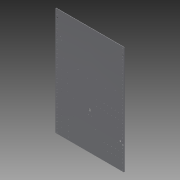
# Autodesk Inventor part: Electronics plate
Saved by Autodesk Inventor 2015 (Build 190159000, 159)
## iProperties
Created: 2015-01-17
Part Number: Electronics plate
Material: Generic
Document SubType Name: Modeling
Designer: chapale16
Density: 1 g/cm^3
Appearance: Default
Author: chapale16
Autodesk Inventor part; units mm, degrees
ref_plane "YZ Plane" through (0, 0, 0) normal (1, 0, 0) x (0, 1, 0)
ref_plane "XZ Plane" through (0, 0, 0) normal (0, 1, 0) x (-1, 0, 0)
sketch "Sketch2" plane through (0, 0, 0) normal (0, 0, 1) x (1, 0, 0)
  line L0 (0, 0) -> (566.42, 0)
  line L1 (566.42, 0) -> (566.42, -1727.2)
  line L2 (566.42, -1727.2) -> (0, -1727.2)
  line L3 (0, -1727.2) -> (0, 0)
  dimension "d0" = 566.42
  dimension "d1" = 1727.2
  constraints: 8 end point, 2 parallel, 1 horizontal, 1 perpendicular
  measures "d0" distance of L1.end L2.end
  measures "d1" distance of L0.end L1.end
extrude "Extrusion1" add sketch "Sketch2" along normal blind 3.175
sketch "Sketch4" plane through (0, 0, 3.175) normal (0, 0, 1) x (1, 0, 0)
  line L0 (566.42, 0) -> (0, 0) projected
  line L1 (0, 0) -> (0, -1727.2) projected
  line L2 (0, -1727.2) -> (566.42, -1727.2) projected
  line L3 (566.42, -1727.2) -> (566.42, 0) projected
  line L4 (0, -1727.2) -> (566.42, -1727.2) projected
  line L5 (68.58, -1727.2) -> (500.38, -1727.2)
  circle A0 centre (68.58, -1391.92) radius 12.7
  circle A1 centre (500.38, -1391.92) radius 12.7
  circle A2 centre (68.58, -1727.2) radius 12.7
  circle A3 centre (500.38, -1727.2) radius 12.7
  dimension "d6" = 25.4
  dimension "d7" = 25.4
  dimension "d8" = 25.4
  dimension "d9" = 25.4
  constraints: 4 centre point, 2 coincident, 2 end point, 1 horizontal, 1 point on line
  measures "d6" diameter of A0
  measures "d7" diameter of A1
  measures "d8" diameter of A2
  measures "d9" diameter of A3
extrude "Extrusion2" add sketch "Sketch4" along normal blind 3.175 contours A0 | A1
sketch "Sketch6" plane through (0, 0, 3.175) normal (0, 0, 1) x (1, 0, 0)
  circle A0 centre (12.7, -1460.5) radius 3.175 projected
  circle A1 centre (553.72, -1460.5) radius 3.175 projected
  circle A2 centre (553.72, -1460.5) radius 4.7625
  circle A3 centre (12.7, -1460.5) radius 4.7625
  point P0 (0, 0)
  dimension "d16" = 9.525
  dimension "d17" = 9.525
  constraints: 2 centre point, 2 coincident
  measures "d16" diameter of A2
  measures "d17" diameter of A3
extrude "Extrusion4" cut sketch "Sketch6" against normal through all contours A0 | A1 | A2 | A3
sketch "Sketch7" plane through (0, 0, 3.175) normal (0, 0, 1) x (1, 0, 0)
  circle A0 centre (12.7, -1460.5) radius 4.7625 projected
  circle A1 centre (12.7, -1460.5) radius 6.35
  circle A2 centre (553.72, -1460.5) radius 4.7625 projected
  circle A3 centre (553.72, -1460.5) radius 6.35
  point P0 (0, 0)
  dimension "d20" = 12.7
  dimension "d21" = 12.7
  constraints: 2 centre point, 2 coincident
  measures "d20" diameter of A1
  measures "d21" diameter of A3
extrude "Extrusion5" cut sketch "Sketch7" against normal blind 12.7 contours A3
sketch "Sketch9" plane through (0, 0, 3.175) normal (0, 0, 1) x (1, 0, 0)
  circle A0 centre (553.72, -825.5) radius 6.35 projected
  circle A1 centre (12.7, -825.5) radius 6.35 projected
  circle A2 centre (12.7, -825.5) radius 6.35
  circle A3 centre (553.72, -825.5) radius 6.35
  point P0 (0, 0)
  constraints: 2 centre point, 2 coincident, 2 concentric
extrude "Extrusion7" cut sketch "Sketch9" against normal blind 3.175
sketch "Sketch10" plane through (0, 0, 3.175) normal (0, 0, 1) x (1, 0, 0)
  line L0 (566.42, 0) -> (566.42, -1727.2) projected
  line L1 (0, -1732.8892) -> (566.42, -1732.8892)
  line L2 (566.42, -1732.8892) -> (566.42, -1054.0894)
  line L3 (566.42, -1054.0894) -> (0, -1054.0894)
  line L4 (0, -1054.0894) -> (0, -1732.8892)
  point P0 (0, 0)
  constraints: 8 end point, 2 parallel, 1 horizontal, 1 perpendicular, 1 point on line
extrude "Extrusion8" cut sketch "Sketch10" along normal blind 25.4
sketch "Sketch13" plane through (0, 0, 3.175) normal (0, 0, 1) x (1, 0, 0)
  line L0 (566.42, -1727.2) -> (566.42, 0) projected
  line L1 (0, 0) -> (566.42, 0)
  line L2 (566.42, 0) -> (566.42, -762)
  line L3 (566.42, -762) -> (0, -762)
  line L4 (0, -762) -> (0, 0)
  dimension "d204" = 762
  constraints: 8 end point, 2 parallel, 1 horizontal, 1 perpendicular, 1 point on line
  measures "d204" distance of L3.end L1.start
extrude "Extrusion10" cut sketch "Sketch13" against normal blind 25.4
hole "Hole1" at (12.7, -1714.5, 3.175) direction (0, 0, -1) diameter 6.35 end through all
pattern_linear "Rectangular Pattern1" count 38 spacing 25.4 along (0, 1, 0) of "Hole1"
hole "Hole2" at (553.72, -1714.5, 3.175) direction (0, 0, -1) diameter 6.35 end through all
pattern_linear "Rectangular Pattern2" count 38 spacing 25.4 along (0, 1, 0) of "Hole2"
ref_plane "Work Plane1" through (283.21, -1727.2, 0) normal (-1, 0, 0) x (0, 0, 1)
sketch "Sketch22" plane through (0, 0, 3.175) normal (0, 0, 1) x (1, 0, 0)
  line L0 (566.42, -1727.2) -> (0, -1727.2) projected
  line L1 (330.2, -1727.2) -> (330.2, -1460.5)
  line L2 (0, -1727.2) -> (0, -762) projected
  circle A0 centre (330.2, -1460.5) radius 2.7781
  line L3 (330.2, -1460.5) -> (512.4704, -1460.5)
  circle A1 centre (512.4704, -1460.5) radius 2.7781
  line L4 (330.2, -1460.5) -> (330.2, -1356.106)
  circle A2 centre (330.2, -1356.106) radius 2.7781
  line L5 (330.2, -1356.106) -> (512.4704, -1356.106)
  circle A3 centre (512.4704, -1356.106) radius 2.7781
  point P0 (0, 0)
  dimension "d145" = 266.7
  dimension "d146" = 330.2
  dimension "d147" = 5.5563
  dimension "d148" = 182.2704
  dimension "d149" = 5.5563
  dimension "d150" = 104.394
  dimension "d151" = 5.5563
  dimension "d152" = 5.5563
  constraints: 8 end point, 4 centre point, 4 coincident, 2 horizontal, 2 parallel, 2 point on line
  measures "d145" distance of L1.start L1.end
  measures "d146" distance between parallel lines of L2 L1
  measures "d147" diameter of A0
  measures "d148" distance of L3.start L3.end
  measures "d149" diameter of A1
  measures "d150" distance of L3.start L4.end
  measures "d151" diameter of A2
  measures "d152" diameter of A3
extrude "Extrusion18" cut sketch "Sketch22" against normal through all
sketch "Sketch24" plane through (0, 0, 3.175) normal (0, 0, 1) x (1, 0, 0)
  line L0 (566.42, -1727.2) -> (0, -1727.2) projected
  line L1 (152.4, -1727.2) -> (152.4, -1460.5)
  line L2 (566.42, -1727.2) -> (566.42, -762) projected
  circle A0 centre (152.4, -1460.5) radius 1.1906
  line L3 (152.4, -1460.5) -> (50.8, -1460.5)
  circle A1 centre (50.8, -1460.5) radius 1.1906
  line L4 (101.6, -1460.5) -> (101.6, -1397)
  line L5 (81.7293, -1397) -> (121.4707, -1397)
  circle A2 centre (152.4, -1333.5) radius 1.1906
  circle A3 centre (50.8, -1333.5) radius 1.1906
  point P0 (0, 0)
  dimension "d166" = 266.7
  dimension "d168" = 2.3813
  dimension "d169" = 101.6
  dimension "d170" = 2.3813
  dimension "d171" = 63.5
  dimension "d242" = 152.4
  constraints: 8 end point, 4 centre point, 2 coincident, 2 horizontal, 2 midpoint, 2 symmetric about line, 2 vertical, 1 point on line, 2 other
  measures "d166" distance of L1.start L1.end
  measures "d168" diameter of A0
  measures "d169" distance of L3.start L3.end
  measures "d170" diameter of A1
  measures "d171" distance of L4.start L4.end
  measures "d242" distance of L1.start L0.end
extrude "Extrusion20" cut sketch "Sketch24" against normal through all
sketch "Sketch25" plane through (0, 0, 3.175) normal (0, 0, 1) x (1, 0, 0)
  line L0 (0, -1727.2) -> (566.42, -1727.2) projected
  line L1 (50.8, -1727.2) -> (50.8, -1308.1)
  line L2 (0, -762) -> (0, -1727.2) projected
  circle A0 centre (50.8, -1308.1) radius 1.9844
  line L3 (50.8, -1308.1) -> (99.6442, -1308.1)
  circle A1 centre (99.6442, -1308.1) radius 1.9844
  line L4 (75.2221, -1308.1) -> (75.2221, -1277.5819)
  line L5 (75.2221, -1277.5819) -> (54.2596, -1277.5819)
  circle A2 centre (50.8, -1247.0638) radius 1.9844
  circle A3 centre (99.6442, -1247.0638) radius 1.9844
  point P0 (0, 0)
  dimension "d174" = 419.1
  dimension "d175" = 50.8
  dimension "d176" = 3.9688
  dimension "d177" = 48.8442
  dimension "d178" = 3.9688
  dimension "d179" = 30.5181
  constraints: 8 end point, 4 centre point, 2 coincident, 2 symmetric about line, 2 vertical, 1 horizontal, 1 midpoint, 1 perpendicular, 1 point on line, 2 other
  measures "d174" distance of L1.start L1.end
  measures "d175" distance between parallel lines of L2 L1
  measures "d176" diameter of A0
  measures "d177" distance of L3.start L3.end
  measures "d178" diameter of A1
  measures "d179" distance of L4.start L4.end
extrude "Extrusion21" cut sketch "Sketch25" against normal through all
sketch "Sketch26" plane through (0, 0, 3.175) normal (0, 0, 1) x (1, 0, 0)
  line L0 (566.42, -1727.2) -> (490.22, -1727.2)
  line L1 (566.42, -1727.2) -> (0, -1727.2) projected
  line L2 (490.22, -1727.2) -> (490.22, -1104.9)
  circle A0 centre (490.22, -1104.9) radius 2.5797
  circle A1 centre (337.82, -1104.9) radius 2.5797
  circle A2 centre (185.42, -1104.9) radius 2.5797
  line L3 (490.22, -1104.9) -> (490.22, -1130.3)
  line L4 (490.22, -1130.3) -> (414.02, -1130.3)
  circle A3 centre (414.02, -1130.3) radius 2.5797
  circle A4 centre (261.62, -1130.3) radius 2.5797
  point P0 (0, 0)
  dimension "d182" = 76.2
  dimension "d183" = 622.3
  dimension "d184" = 5.1594
  dimension "d187" = 152.4
  dimension "d192" = 25.4
  dimension "d193" = 76.2
  dimension "d194" = 5.1594
  dimension "d197" = 152.4
  constraints: 8 end point, 5 centre point, 4 coincident, 3 horizontal, 2 point on line, 1 perpendicular, 8 other
  measures "d182" distance of L0.start L0.end
  measures "d183" distance of L0.end L2.end
  measures "d184" diameter of A0
  measures "d187" distance of L2.end point (337.82, -1104.9)
  measures "d192" distance of L3.start L3.end
  measures "d193" distance of L3.end L4.end
  measures "d194" diameter of A3
  measures "d197" distance of A3.centre A4.centre
extrude "Extrusion22" cut sketch "Sketch26" against normal through all
sketch "Sketch29" plane through (0, 0, 3.175) normal (0, 0, 1) x (1, 0, 0)
  line L0 (0, -1727.2) -> (566.42, -1727.2) projected
  line L1 (50.8, -1727.2) -> (50.8, -1625.6)
  line L2 (0, -762) -> (0, -1727.2) projected
  circle A0 centre (50.8, -1625.6) radius 2.5797
  line L3 (50.8, -1625.6) -> (109.5, -1625.6)
  circle A1 centre (109.5, -1625.6) radius 2.5797
  point P0 (0, 0)
  dimension "d233" = 101.6
  dimension "d234" = 90
  dimension "d236" = 50.8
  dimension "d237" = 5.1594
  dimension "d238" = 58.7
  dimension "d239" = 5.1594
  dimension "d293" = 90
  constraints: 4 end point, 2 centre point, 2 coincident, 1 point on line
  measures "d233" distance of L1.start L1.end
  measures "d234" angle of L0 L1
  measures "d236" distance from line of L1.start L2
  measures "d237" diameter of A0
  measures "d238" distance of L3.start L3.end
  measures "d239" diameter of A1
  measures "d293" angle of L1 L3
extrude "Extrusion25" cut sketch "Sketch29" against normal through all
sketch "Sketch30" plane through (0, 0, 3.175) normal (0, 0, 1) x (1, 0, 0)
  line L0 (0, -762) -> (63.5, -762)
  line L1 (63.5, -762) -> (63.5, -1092.2)
  line L2 (63.5, -1092.2) -> (0, -1092.2)
  line L3 (0, -1092.2) -> (0, -762)
  circle A0 centre (63.5, -1092.2) radius 1.5875
  line L4 (63.5, -1092.2) -> (90.5002, -1092.2)
  circle A1 centre (90.5002, -1092.2) radius 1.5875
  point P0 (0, 0)
  dimension "d243" = 63.5
  dimension "d244" = 330.2
  dimension "d245" = 3.175
  dimension "d246" = 27.0002
  dimension "d247" = 3.175
  dimension "d291" = 90
  constraints: 10 end point, 2 centre point, 2 coincident, 2 parallel, 1 horizontal, 1 perpendicular
  measures "d243" distance of L1.end L2.end
  measures "d244" distance of L0.end L1.end
  measures "d245" diameter of A0
  measures "d246" distance of L4.start L4.end
  measures "d247" diameter of A1
  measures "d291" angle of L4 L1
extrude "Extrusion26" cut sketch "Sketch30" against normal through all contours A1 | A0 L4 L1 | L1 L2 A0 | L2 L4 A0
sketch "Sketch31" plane through (0, 0, 3.175) normal (0, 0, 1) x (1, 0, 0)
  line L0 (566.42, -1727.2) -> (566.42, -762) projected
  line L1 (0, -1727.2) -> (566.42, -1727.2)
  line L2 (566.42, -1727.2) -> (566.42, -1651)
  line L3 (566.42, -1651) -> (0, -1651)
  line L4 (0, -1651) -> (0, -1727.2)
  point P0 (0, 0)
  dimension "d259" = 76.2
  constraints: 8 end point, 2 parallel, 1 horizontal, 1 perpendicular, 1 point on line
  measures "d259" distance between parallel lines of L1 L3
extrude "Extrusion27" cut sketch "Sketch31" against normal through all
sketch "Sketch32" plane through (0, 0, 3.175) normal (0, 0, 1) x (1, 0, 0)
  line L0 (0, -1651) -> (0, -762) projected
  line L1 (566.42, -1651) -> (0, -1651) projected
  line L2 (0, -1244.6) -> (520.7, -1244.6)
  line L3 (520.7, -1244.6) -> (520.7, -1651)
  line L4 (520.7, -1651) -> (0, -1651)
  line L5 (0, -1651) -> (0, -1244.6)
  circle A0 centre (520.7, -1244.6) radius 2.5797
  line L6 (520.7, -1244.6) -> (520.7, -1295.4)
  circle A1 centre (520.7, -1295.4) radius 2.5797
  point P0 (0, 0)
  dimension "d262" = 520.7
  dimension "d263" = 406.4
  dimension "d264" = 5.1594
  dimension "d265" = 50.8
  dimension "d266" = 5.1594
  constraints: 10 end point, 3 point on line, 2 centre point, 2 coincident, 2 parallel, 1 horizontal, 1 perpendicular
  measures "d262" distance of L0.start L3.end
  measures "d263" distance between parallel lines of L1 L2
  measures "d264" diameter of A0
  measures "d265" distance of L6.start L6.end
  measures "d266" diameter of A1
extrude "Extrusion28" cut sketch "Sketch32" against normal through all contours A0 L3 L2 | L2 L3 A0 | A1 L3 | L3 A1
sketch "Sketch37" plane through (0, 0, 3.175) normal (0, 0, 1) x (1, 0, 0)
  line L0 (0, -1651) -> (0, -762) projected
  line L1 (566.42, -1651) -> (0, -1651) projected
  line L2 (50.8, -1651) -> (50.8, -965.2)
  line L3 (50.8, -965.2) -> (0, -965.2)
  circle A0 centre (50.8, -965.2) radius 2.7781
  line L4 (50.8, -965.2) -> (50.8, -941.705)
  line L5 (50.8, -941.705) -> (42.799, -941.705)
  line L6 (42.799, -941.705) -> (42.799, -965.2)
  line L7 (42.799, -965.2) -> (50.8, -965.2)
  circle A1 centre (42.799, -941.705) radius 2.7781
  point P0 (0, 0)
  dimension "d283" = 50.8
  dimension "d284" = 685.8
  dimension "d285" = 5.5563
  dimension "d286" = 23.495
  dimension "d287" = 8.001
  dimension "d288" = 5.5563
  dimension "d292" = 180
  constraints: 12 end point, 2 centre point, 2 coincident, 2 parallel, 2 perpendicular, 2 point on line, 1 vertical
  measures "d283" distance of L2.end L3.end
  measures "d284" distance of L2.start L2.end
  measures "d285" diameter of A0
  measures "d286" distance of L4.start L4.end
  measures "d287" distance of L4.end L5.end
  measures "d288" diameter of A1
  measures "d292" angle of L2 L4
extrude "Extrusion32" cut sketch "Sketch37" against normal through all contours A0 L3 L2 | L2 L4 A0 | A0 L4 L3 | A1 L5 L6 | L6 L5 A1
pattern_linear "Rectangular Pattern9" count 7 spacing 30.48 along (-1, 0, 0) count 2 spacing 273.05 along (0, -1, 0) of "Extrusion28"
sketch "Sketch38" plane through (0, 0, 3.175) normal (0, 0, 1) x (1, 0, 0)
  line L0 (322.6238, -1480.7724) -> (377.7515, -1480.7724)
  line L1 (377.7515, -1480.7724) -> (377.7515, -1593.1826)
  line L2 (377.7515, -1593.1826) -> (322.6238, -1593.1826)
  line L3 (322.6238, -1593.1826) -> (322.6238, -1480.7724)
  point P0 (0, 0)
  constraints: 8 end point, 2 parallel, 1 horizontal, 1 perpendicular
extrude "Extrusion33" add sketch "Sketch38" against normal blind 3.175
sketch "Sketch39" plane through (0, 0, 3.175) normal (0, 0, 1) x (1, 0, 0)
  line L0 (0, -1651) -> (566.42, -1651) projected
  line L1 (50.8, -1651) -> (50.8, -1219.2)
  line L2 (0, -762) -> (0, -1651) projected
  circle A0 centre (50.8, -1219.2) radius 1.9844
  line L3 (50.8, -1219.2) -> (98.552, -1219.2)
  line L4 (98.552, -1219.2) -> (98.552, -1176.147)
  line L5 (98.552, -1176.147) -> (50.8, -1176.147)
  line L6 (50.8, -1176.147) -> (50.8, -1219.2)
  circle A1 centre (98.552, -1176.147) radius 1.9844
  circle A2 centre (50.8, -1176.147) radius 1.9844
  circle A3 centre (98.552, -1219.2) radius 1.9844
  point P0 (0, 0)
  dimension "d305" = 50.8
  dimension "d306" = 431.8
  dimension "d307" = 3.9688
  dimension "d308" = 47.752
  dimension "d309" = 43.053
  dimension "d310" = 3.9688
  dimension "d311" = 3.9688
  dimension "d312" = 3.9688
  constraints: 10 end point, 4 centre point, 4 coincident, 2 parallel, 1 horizontal, 1 perpendicular, 1 point on line, 1 vertical
  measures "d305" distance between parallel lines of L2 L1
  measures "d306" distance of L1.start L1.end
  measures "d307" diameter of A0
  measures "d308" distance of L3.start L3.end
  measures "d309" distance of L3.end L4.end
  measures "d310" diameter of A1
  measures "d311" diameter of A2
  measures "d312" diameter of A3
extrude "Extrusion34" cut sketch "Sketch39" against normal blind 3.175 contours A0 L6 L1 | L1 L3 A0 | L6 A0 L3 | A2 L5 L6 | L6 L5 A2 | A3 L4 L3 | L3 L4 A3 | A1 L4 L5 | L5 L4 A1
sketch "Sketch41" plane through (0, 0, 3.175) normal (0, 0, 1) x (1, 0, 0)
  line L0 (0, -1651) -> (283.21, -1651)
  line L1 (283.21, -1651) -> (283.21, -1346.2)
  line L2 (283.21, -1346.2) -> (0, -1346.2)
  line L3 (0, -1346.2) -> (0, -1651)
  circle A0 centre (283.21, -1346.2) radius 11.1125
  point P0 (0, 0)
  dimension "d325" = 22.225
  dimension "d328" = 283.21
  dimension "d329" = 304.8
  constraints: 8 end point, 2 parallel, 1 centre point, 1 coincident, 1 horizontal, 1 perpendicular
  measures "d325" diameter of A0
  measures "d328" distance of L0.start L0.end
  measures "d329" distance of L2.end L0.start
extrude "Extrusion36" cut sketch "Sketch41" against normal blind 25.4 contours A0 L2 L1 | L1 L2 A0
sketch "Sketch42" plane through (0, 0, 3.175) normal (0, 0, 1) x (1, 0, 0)
  line L0 (566.42, -1651) -> (532.003, -1651)
  line L1 (532.003, -1651) -> (532.003, -1443.99)
  line L2 (532.003, -1443.99) -> (566.42, -1443.99)
  line L3 (566.42, -1443.99) -> (566.42, -1651)
  circle A0 centre (532.003, -1443.99) radius 7.62
  point P0 (0, 0)
  dimension "d330" = 15.24
  dimension "d333" = 207.01
  constraints: 8 end point, 2 parallel, 1 centre point, 1 coincident, 1 horizontal, 1 perpendicular
  measures "d330" diameter of A0
  measures "d333" distance of L2.end L0.start
extrude "Extrusion37" cut sketch "Sketch42" against normal through all contours A0 L2 L1 | L1 L2 A0
pattern_linear "Rectangular Pattern12" count 4 spacing 41.783 along (0, 1, 0) of "Extrusion25"
sketch "Sketch43" plane through (0, 0, 3.175) normal (0, 0, 1) x (1, 0, 0)
  circle A0 centre (283.21, -1346.2) radius 11.1125 projected
  line L0 (283.21, -1346.2) -> (283.21, -1384.3)
  line L1 (283.21, -1384.3) -> (273.685, -1384.3)
  line L2 (273.685, -1384.3) -> (292.735, -1384.3)
  circle A1 centre (273.685, -1384.3) radius 3.175
  circle A2 centre (292.735, -1384.3) radius 3.175
  point P0 (0, 0)
  dimension "d337" = 38.1
  dimension "d338" = 9.525
  dimension "d339" = 19.05
  dimension "d340" = 6.35
  dimension "d341" = 6.35
  constraints: 6 end point, 2 centre point, 2 coincident, 1 perpendicular, 1 point on line, 1 vertical
  measures "d337" distance of L0.start L0.end
  measures "d338" distance of L0.end L1.end
  measures "d339" distance of L1.end L2.end
  measures "d340" diameter of A1
  measures "d341" diameter of A2
extrude "Extrusion38" cut sketch "Sketch43" against normal through all contours A2 | A1
fillet "Fillet1" radius 6.35 4 edges at (566.42, -762, 1.5875) (0, -762, 1.5875) (0, -1651, 1.5875) (566.42, -1651, 1.5875)
equation "\"d22\" = d20"
body "Solid1"
